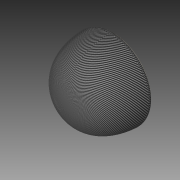
# Autodesk Inventor part: Headlight_Round_Body
Saved by Autodesk Inventor 2016 (Build 200138000, 138)
## iProperties
Created: 2015-08-10
Part Number: Headlight_Round_Body
Material: Generic
Document SubType Name: Modeling
Designer: Yann
Density: 1 g/cm^3
Appearance: Default
Author: Yann
Autodesk Inventor part; units mm, degrees
ref_plane "YZ Plane" through (0, 0, 0) normal (1, 0, 0) x (0, 1, 0)
ref_plane "XZ Plane" through (0, 0, 0) normal (0, 1, 0) x (-1, 0, 0)
ref_plane "XY Plane" through (0, 0, 0) normal (0, 0, 1) x (1, 0, 0)
sketch "Sketch1" plane through (0, 0, 0) normal (1, 0, 0) x (0, 1, 0)
  line L0 (0, 83.005) -> (-53.7025, 83.005) construction
  line L1 (-53.7025, 83.005) -> (-102.16, 61.497) construction
  line L2 (-102.16, 61.497) -> (-102.16, 0) construction
  spline S0 degree 3 poles (0, 83.005) (-53.7025, 83.005) (-102.16, 61.497) (-102.16, 0) knots 1 1 1 1 2 2 2 2
  line L3 (0, 130.2378) -> (0, -22.9579) construction
  line L4 (-149.6326, 0) -> (28.7335, 0) construction
  line L5 (0, 0) -> (0, 83.005)
  line L6 (0, 0) -> (-102.16, 0)
  dimension "d0" = 102.16
  dimension "d1" = 83.005
  constraints: 4 end point, 2 collinear, 2 point on line, 1 horizontal, 1 vertical, 3 other
  measures "d0" distance of L5.start L2.end
  measures "d1" distance from line of L4 L0.start
revolve "Revolution1" add sketch "Sketch1" angle 360 about axis through (0, 0, 0) along (0, 1, 0)
fillet "Fillet1" radius 10 1 edges at (0, 0, -83.005)
sketch "Sketch2" plane through (0.0005, 0, -0.0146) normal (0, 1, 0) x (1, 0, 0)
  line L0 (-81.5447, 81.5295) -> (81.7711, 81.5295) construction
  line L1 (81.7711, 81.5295) -> (81.7711, -81.0807) construction
  line L2 (81.7711, -81.0807) -> (-81.5447, -81.0807) construction
  line L3 (-81.5447, -81.0807) -> (-81.5447, 81.5295) construction
  point P0 (-0.0005, -0.0146)
  constraints: 2 other
decal "Decal1"
body "Solid1"
